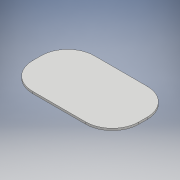
# Autodesk Inventor part: Game_Colonies
Saved by Autodesk Inventor 2018 (Build 220112000, 112)
## iProperties
Created: 2021-04-21
Part Number: Game_Colonies
Material: Generic
Document SubType Name: Modeling
Designer: Bradley
Density: 1 g/cm^3
Appearance: Default
Author: Bradley
Autodesk Inventor part; units mm, degrees
ref_plane "YZ Plane" through (0, 0, 0) normal (1, 0, 0) x (0, 1, 0)
ref_plane "XZ Plane" through (0, 0, 0) normal (0, 1, 0) x (-1, 0, 0)
ref_plane "XY Plane" through (0, 0, 0) normal (0, 0, 1) x (1, 0, 0)
sketch "Sketch1" plane through (0, 0, 0) normal (0, 0, 1) x (1, 0, 0)
  line L0 (-25, -29) -> (25, -29)
  line L1 (50, -4) -> (50, 4)
  line L2 (25, 29) -> (-25, 29)
  line L3 (-50, 4) -> (-50, -4)
  line L4 (-50, -29) -> (50, 29) construction
  line L5 (50, -29) -> (-50, 29) construction
  arc A0 (50, 4) -> (25, 29) centre (25, 4) ccw
  arc A1 (25, -29) -> (50, -4) centre (25, -4) ccw
  arc A2 (-50, -4) -> (-25, -29) centre (-25, -4) ccw
  arc A3 (-25, 29) -> (-50, 4) centre (-25, 4) ccw
  point P0 (0, 0)
  dimension "d0" = 100
  dimension "d1" = 58
  dimension "d2" = 25
  constraints: 12 end point, 8 point on circle, 8 point on line, 8 tangent, 4 centre point, 3 equal radius, 2 midpoint, 2 parallel, 1 horizontal, 1 perpendicular
  measures "d0" distance of L5.end L4.end
  measures "d1" distance of L4.end L5.start
  measures "d2" radius of A0
extrude "Extrusion1" add sketch "Sketch1" along normal mid plane 1.93
body "Solid1"
